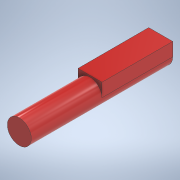
# Autodesk Inventor part: Sensor
Saved by Autodesk Inventor 2021 (Build 250183000, 183)
## iProperties
Created: 2021-03-30
Part Number: Sensor
Material: Generic
Document SubType Name: Modeling
Designer: Darek
Density: 1 g/cm^3
Appearance: Default
Author: Darek
Autodesk Inventor part; units mm, degrees
ref_plane "YZ Plane" through (0, 0, 0) normal (1, 0, 0) x (0, 1, 0)
ref_plane "XZ Plane" through (0, 0, 0) normal (0, 1, 0) x (-1, 0, 0)
ref_plane "XY Plane" through (0, 0, 0) normal (0, 0, 1) x (1, 0, 0)
sketch "Sketch1" plane through (0, 0, 0) normal (0, 0, 1) x (1, 0, 0)
  circle A0 centre (0, 0) radius 1.6964
  line L0 (0, 0) -> (1.6964, 0)
  line L1 (1.6964, 0) -> (1.6964, 1.8999)
  line L2 (1.6964, 1.8999) -> (0, 1.8999)
  line L3 (0, 1.8999) -> (0, 0)
  line L4 (0, 0) -> (-1.6964, 0)
  line L5 (-1.6964, 0) -> (-1.6964, 1.8999)
  line L6 (-1.6964, 1.8999) -> (0, 1.8999)
  line L7 (0, 1.8999) -> (0, 0)
  point P0 (0, 1.6964)
  constraints: 16 end point, 4 parallel, 2 horizontal, 2 perpendicular, 1 centre point, 1 coincident, 1 point on line
extrude "Extrusion1" add sketch "Sketch1" along normal blind 20 contours L4 L0 A0 | A0 L3 L4 | L0 L3 A0
extrude "Extrusion2" add sketch "Sketch1" along normal blind 10 contours L5 L6 L3 A0 | A0 L3 L2 L1
body "Solid1"
